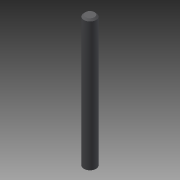
# Autodesk Inventor part: 2838_pin
Saved by Autodesk Inventor 2014 SP2 (Build 180246200, 246)
## iProperties
Created: 2018-07-20
Part Number: 2838_pin
Material: Generic
Catalog Web Link: www.cadenas.de
Description: 2830, 2831, 2832, 2833, 2835, 2836, 2837, 2838, 2839, 2840, 2841, 2842_pin-Economy Lift-Off Hinges
Vendor: 8020
Document SubType Name: Modeling
Designer: psadmin
Manufacturer: 8020
Mass: 0.897388 g
Surface Area: 7.87397 cm^2
Volume: 0.897388 cm^3
Density: 1 g/cm^3
Appearance: PSOLRGB-127-127-127
Category: PARTsolutions
Company: 8020
Title: 2838_pin
Author: Cadenas PARTsolutions
Comments: Economy Lift-Off Hinges
PSOL_IDENT_0: {$CADENAS_DATA\23d-libs\8020\inch\panels_and_doors\2830_pin.prj},228 {VTYP=3D},{NB=2838_pin},{LINA=2
PSOL_IDENT_1: 838_pin},{NN=2830, 2831, 2832, 2833, 2835, 2836, 2837, 2838, 2839, 2840, 2841, 2842_pin},{DATE=16.03
PSOL_IDENT_2: .2018 08:23:49},{GEOMDATE=08.02.2012 08:44:00},{VERSION=},{LINEID=10},{WBVAR=TYPE},{WBNUMERIC=}  {NB=
PSOL_IDENT_3: 2838_pin},{LINA=2838_pin},{KT=DUMMY},{PN=2838},{SERIES=10 Series},{TYPE=5},{MAT=Aluminum},{FIN=Clear
PSOL_IDENT_4: Anodize},{A=2.000},{H=0.187},{L=1.000},{NO=8},{L1=1}
NN: 2830, 2831, 2832, 2833, 2835, 2836, 2837, 2838, 2839, 2840, 2841, 2842_pin
NT: Economy Lift-Off Hinges
NB: 2838_pin
NBSYN: $PN._pin
LINA: 2838_pin
SERIES: 10 Series
TYPE: Right Hinge Long Pin
MAT: Aluminum
FIN: Clear Anodize
A: 2
H: 0.187
SUPPLIER: 8020
ARTICLENO: 2838_pin
BOMINFO: 2838_pin
CREATOR: CADENAS GmbH
Autodesk Inventor part; units mm, degrees
sketch "Sketch_1" plane through (0, 0, 0) normal (0, 0, 1) x (1, 0, 0)
  line L0 (0, 0) -> (0, 50.8)
  line L1 (0, 50.8) -> (1.7399, 50.8)
  line L2 (1.7399, 50.8) -> (2.3749, 50.165)
  line L3 (2.3749, 50.165) -> (2.3749, 0)
  line L4 (2.3749, 0) -> (0, 0)
  line L5 (0, 0) -> (0, 50.8)
  constraints: 12 end point
revolve "Revolution1" add sketch "Sketch_1" angle 360 about axis through (0, 0, 0) along (0, -1, 0)
ref_plane "to_left_XY" through (0, 0, 0) normal (0, 1, 0) x (1, 0, 0)
ref_plane "to_left_YZ" through (0, 0, 0) normal (1, 0, 0) x (0, 0, -1)
ref_plane "to_left_ZX" through (0, 0, 0) normal (0, 0, -1) x (0, 1, 0)
body "Solid1"
